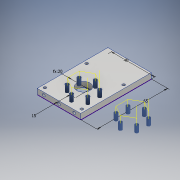
# Autodesk Inventor part: wheel_fix_plate_collet
Saved by Autodesk Inventor 2018 (Build 220112000, 112)
## iProperties
Created: 2017-08-19
Part Number: wheel_fix_plate_collet
Material: Aluminum 6061
Document SubType Name: Modeling
Designer: steve
Density: 2.7 g/cm^3
Appearance: Aluminum - Flat
Mass: 48.6491 g
Surface Area: 67.3624 cm^2
Volume: 18.0182 cm^3
Author: steve
Autodesk Inventor part; units mm, degrees
ref_plane "YZ Plane" through (0, 0, 0) normal (1, 0, 0) x (0, 1, 0)
ref_plane "XZ Plane" through (0, 0, 0) normal (0, 1, 0) x (-1, 0, 0)
ref_plane "XY Plane" through (0, 0, 0) normal (0, 0, 1) x (1, 0, 0)
sketch "Sketch1" plane through (0, 0, 0) normal (0, 0, 1) x (1, 0, 0)
  line L0 (20, -15) -> (-20, -15)
  line L1 (-20, -15) -> (-20, 50)
  line L2 (-20, 50) -> (20, 50)
  line L3 (20, 50) -> (20, -15)
  point P0 (0, 0)
  dimension "d0" = 40
  dimension "d1" = 65
  dimension "d27" = 15
  dimension "d28" = 20
  constraints: 8 end point, 2 parallel, 1 horizontal, 1 perpendicular
  measures "d0" distance of L1.end L2.end
  measures "d1" distance of L2.end L0.start
  measures "d27" distance from line of L0 point (0, 0)
  measures "d28" distance from line of L1 point (0, 0)
extrude "Extrusion1" add sketch "Sketch1" along normal blind 5
sketch "Sketch5" plane through (-20, -15, 0) normal (0, -1, 0) x (1, 0, 0)
  line L0 (20, 0) -> (20, 7.6333) construction
  line L1 (0, 0) -> (0, 5) construction
  line L2 (0, 2.5) -> (40, 2.5) construction
  line L3 (40, 0) -> (40, 5) construction
  line L4 (20, 0) -> (20, 7.6333) construction
  line L5 (0, 5) -> (40, 5) construction
  point P0 (20, 2.5)
  point P1 (6, 2.5)
  point P2 (34, 2.5)
  dimension "d29" = 14
  constraints: 6 end point, 3 midpoint, 1 perpendicular, 1 point on line, 1 symmetric about line
  measures "d29" distance of point (20, 2.5) point (6, 2.5)
hole "Hole3" at (0, -15, 2.5) at (-14, -15, 2.5) at (14, -15, 2.5) direction (0, 1, 0) diameter 2.459 depth 8.8 tip angle 118 thread size "M3x0.5" class "6H" standard "ISO Metric profile"
sketch "Sketch6" plane through (0, 0, 5) normal (0, 0, 1) x (1, 0, 0)
  line L0 (-39.4918, 7.5) -> (40.0477, 7.5) construction
  line L1 (-20, -15) -> (20, -15) construction
  line L2 (20, -15) -> (20, 50) construction
  line L3 (20, 50) -> (-20, 50) construction
  line L4 (-20, 50) -> (-20, -15) construction
  circle A0 centre (0, 7.5) radius 6.05
  line L5 (0, 63) -> (0, -28) construction
  circle A1 centre (0, 7.5) radius 11 construction
  circle A2 centre (0, -3.5) radius 1.5
  circle A3 centre (9.5263, 2) radius 1.5
  circle A4 centre (9.5263, 13) radius 1.5
  circle A5 centre (0, 18.5) radius 1.5
  circle A6 centre (-9.5263, 13) radius 1.5
  circle A7 centre (-9.5263, 2) radius 1.5
  point P0 (0, 0)
  dimension "d40" = 22
  dimension "d38" = 22.5
  dimension "d39" = 12.1
  dimension "d41" = 3
  dimension "d44" = 360
  constraints: 7 centre point, 3 point on line, 2 end point, 1 coincident, 1 horizontal, 1 vertical alignment, 15 other
  measures "d38" distance between parallel lines of L1 L0
  measures "d39" diameter of A0
  measures "d41" diameter of A2
extrude "Extrusion3" cut sketch "Sketch6" against normal through all
sketch "Sketch7" plane through (0, 0, 5) normal (0, 0, 1) x (1, 0, 0)
  circle A0 centre (0, 7.5) radius 7.05
  circle A1 centre (0, 7.5) radius 6.05 projected
  point P0 (0, 0)
  dimension "d48" = 1
  constraints: 1 centre point, 1 concentric
  measures "d48" radial gap between concentric circles of A1 A0
extrude "Extrusion4" [suppressed]
sketch "Sketch8" plane through (-20, 50, 0) normal (0, 1, 0) x (1, 0, 0)
  circle A0 centre (6, -2.5) radius 1.2295 construction
  circle A1 centre (20, -2.5) radius 1.2295 construction
  circle A2 centre (34, -2.5) radius 1.2295 construction
  point P0 (20, 0)
hole "Hole4" at (14, 50, 2.5) at (0, 50, 2.5) at (-14, 50, 2.5) direction (0, -1, 0) diameter 2.459 depth 8.8 tip angle 118 thread size "M3x0.5" class "6H" standard "ANSI Metric M Profile"
sketch "Sketch9" plane through (0, 0, 5) normal (0, 0, 1) x (1, 0, 0)
  line L0 (17, -11) -> (-17, -11) construction
  line L1 (-17, -11) -> (-17, 27.5) construction
  line L2 (-17, 27.5) -> (17, 27.5) construction
  line L3 (17, 27.5) -> (17, -11) construction
  line L4 (17, -11) -> (-17, 27.5) construction
  line L5 (-17, -11) -> (17, 27.5) construction
  line L6 (-20, -15) -> (20, -15) construction
  line L7 (0, 63) -> (0, -28) construction
  point P0 (0, 0)
  point P1 (0, 8.25)
  dimension "d31" = 6
  dimension "d58" = 34
  dimension "d59" = 38.5
  dimension "d60" = 4
  constraints: 12 end point, 4 coincident, 2 parallel, 1 horizontal, 1 midpoint, 1 perpendicular, 1 point on line
  measures "d58" distance of L1.end L2.end
  measures "d59" distance of L2.end L0.start
  measures "d60" distance between parallel lines of L6 L0
hole "Hole5" at (-17, 27.5, 5) at (17, 27.5, 5) at (17, -11, 5) at (-17, -11, 5) direction (0, 0, -1) diameter 2.5 end through all
equation "\"d28\" = 0.5 * d0"
body "Solid1"
